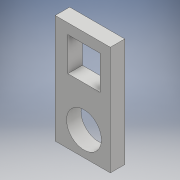
# Autodesk Inventor part: LeadScrewTrackConnection
Saved by Autodesk Inventor 2017 (Build 210142000, 142)
## iProperties
Created: 2016-12-07
Part Number: LeadScrewTrackConnection
Material: Generic
Document SubType Name: Modeling
Designer: umr
Density: 1 g/cm^3
Appearance: Default
Author: umr
Autodesk Inventor part; units mm, degrees
ref_plane "YZ Plane" through (0, 0, 0) normal (1, 0, 0) x (0, 1, 0)
ref_plane "XZ Plane" through (0, 0, 0) normal (0, 1, 0) x (-1, 0, 0)
ref_plane "XY Plane" through (0, 0, 0) normal (0, 0, 1) x (1, 0, 0)
sketch "Sketch1" plane through (0, 0, 0) normal (0, 1, 0) x (-1, 0, 0)
  line L0 (0, 0) -> (38.0445, 0)
  line L1 (38.0445, 0) -> (38.0445, -75.1402)
  line L2 (38.0445, -75.1402) -> (0, -75.1402)
  line L3 (0, -75.1402) -> (0, 0)
  constraints: 8 end point, 2 parallel, 1 horizontal, 1 perpendicular
extrude "Extrusion1" add sketch "Sketch1" along normal blind 10
sketch "Sketch2" plane through (0, 10, 0) normal (0, 1, 0) x (1, 0, 0)
  line L0 (-29.3046, 7.0846) -> (-7.0846, 7.0846)
  line L1 (-7.0846, 7.0846) -> (-7.0846, 30.4317)
  line L2 (-7.0846, 30.4317) -> (-29.3046, 30.4317)
  line L3 (-29.3046, 30.4317) -> (-29.3046, 7.0846)
  circle A0 centre (-18.1946, 58.4482) radius 12.0514
  point P0 (0, 0)
  constraints: 8 end point, 2 parallel, 1 centre point, 1 horizontal, 1 perpendicular
extrude "Extrusion2" cut sketch "Sketch2" against normal up to next
body "Solid1"
